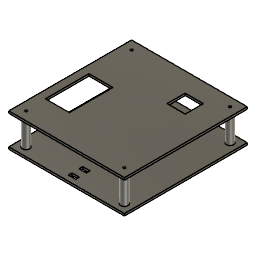
base_colonnine_M3_asole_aperture_superiori_Arduino_pacco_batteria (Autodesk Fusion 360 design; units mm, degrees)
part number: 2026-07-13-17-16-51-748
part number: 2026-07-13-17-16-52-029
part number: 2026-07-13-17-16-52-072
Autodesk Fusion 360 part; units mm, degrees
sketch "Schizzo1" plane through (0, 0, 0) normal (0, 0, 1) x (1, 0, 0) in component "01_Piano_inferiore_con_colonnine_M3"
  line L0 (-80, -85) -> (80, -85)
  line L1 (80, -85) -> (80, 85)
  line L2 (80, 85) -> (-80, 85)
  line L3 (-80, 85) -> (-80, -85)
extrude "Estrusione_Piano_inferiore" add sketch "Schizzo1" along normal blind 3 makes body 1 in component "01_Piano_inferiore_con_colonnine_M3"
ref_plane "Piano di lavoro1" through (0, 0, 43) normal (0, 0, 1) x (1, 0, 0) in component "02_Piano_superiore"
sketch "Schizzo1 (2)" plane through (0, 0, 43) normal (0, 0, 1) x (1, 0, 0) in component "02_Piano_superiore"
  line L0 (-80, -85) -> (80, -85)
  line L1 (80, -85) -> (80, 85)
  line L2 (80, 85) -> (-80, 85)
  line L3 (-80, 85) -> (-80, -85)
extrude "Estrusione_Piano_superiore" add sketch "Schizzo1 (2)" along normal blind 3 separate body makes body 2 in component "02_Piano_superiore"
ref_plane "Piano di lavoro1" through (0, 0, 3) normal (0, 0, 1) x (1, 0, 0) in component "01_Piano_inferiore_con_colonnine_M3"
ref_plane "Piano di lavoro2" through (0, 0, 40.4) normal (0, 0, 1) x (1, 0, 0) in component "01_Piano_inferiore_con_colonnine_M3"
sketch "Schizzo2" plane through (0, 0, 0) normal (0, 0, 1) x (1, 0, 0) in component "01_Piano_inferiore_con_colonnine_M3"
  line L0 (-5, -77.5) -> (5, -77.5)
  line L1 (5, -77.5) -> (5, -72.5)
  line L2 (5, -72.5) -> (-5, -72.5)
  line L3 (-5, -72.5) -> (-5, -77.5)
extrude "Asola_fascetta_01" cut sketch "Schizzo2" along normal blind 3 bodies 1 in component "01_Piano_inferiore_con_colonnine_M3"
sketch "Schizzo3" plane through (0, 0, 0) normal (0, 0, 1) x (1, 0, 0) in component "01_Piano_inferiore_con_colonnine_M3"
  line L0 (-5, -62.5) -> (5, -62.5)
  line L1 (5, -62.5) -> (5, -57.5)
  line L2 (5, -57.5) -> (-5, -57.5)
  line L3 (-5, -57.5) -> (-5, -62.5)
extrude "Asola_fascetta_02" cut sketch "Schizzo3" along normal blind 3 bodies 1 in component "01_Piano_inferiore_con_colonnine_M3"
sketch "Schizzo4" plane through (0, 0, 0) normal (0, 0, 1) x (1, 0, 0) in component "01_Piano_inferiore_con_colonnine_M3"
  line L0 (-5, -12.5) -> (5, -12.5)
  line L1 (5, -12.5) -> (5, -7.5)
  line L2 (5, -7.5) -> (-5, -7.5)
  line L3 (-5, -7.5) -> (-5, -12.5)
extrude "Asola_fascetta_03" cut sketch "Schizzo4" along normal blind 3 bodies 1 in component "01_Piano_inferiore_con_colonnine_M3"
sketch "Schizzo5" plane through (0, 0, 0) normal (0, 0, 1) x (1, 0, 0) in component "01_Piano_inferiore_con_colonnine_M3"
  line L0 (-5, 2.5) -> (5, 2.5)
  line L1 (5, 2.5) -> (5, 7.5)
  line L2 (5, 7.5) -> (-5, 7.5)
  line L3 (-5, 7.5) -> (-5, 2.5)
extrude "Asola_fascetta_04" cut sketch "Schizzo5" along normal blind 3 bodies 1 in component "01_Piano_inferiore_con_colonnine_M3"
sketch "Schizzo2 (2)" plane through (0, 0, 43) normal (0, 0, 1) x (1, 0, 0) in component "02_Piano_superiore"
  circle A0 centre (-68, -73) radius 1.6
extrude "Foro_M3_superiore_01" cut sketch "Schizzo2 (2)" along normal blind 3 bodies 2 in component "02_Piano_superiore"
sketch "Schizzo6" plane through (0, 0, 3) normal (0, 0, 1) x (1, 0, 0) in component "01_Piano_inferiore_con_colonnine_M3"
  circle A0 centre (-68, -73) radius 5
extrude "Estrusione_Colonnina_M3_01" add sketch "Schizzo6" along normal blind 40 bodies 1 in component "01_Piano_inferiore_con_colonnine_M3"
sketch "Schizzo7" plane through (0, 0, 0) normal (0, 0, 1) x (1, 0, 0) in component "01_Piano_inferiore_con_colonnine_M3"
  circle A0 centre (-68, -73) radius 1.6
extrude "Foro_passante_M3_colonnina_01" cut sketch "Schizzo7" along normal blind 43 bodies 1 in component "01_Piano_inferiore_con_colonnine_M3"
sketch "Schizzo8" plane through (0, 0, 40.4) normal (0, 0, 1) x (1, 0, 0) in component "01_Piano_inferiore_con_colonnine_M3"
  line L0 (-65.1, -71.3257) -> (-68, -69.6514)
  line L1 (-68, -69.6514) -> (-70.9, -71.3257)
  line L2 (-70.9, -71.3257) -> (-70.9, -74.6743)
  line L3 (-70.9, -74.6743) -> (-68, -76.3486)
  line L4 (-68, -76.3486) -> (-65.1, -74.6743)
  line L5 (-65.1, -74.6743) -> (-65.1, -71.3257)
extrude "Sede_dado_M3_01" cut sketch "Schizzo8" along normal blind 2.6 bodies 1 in component "01_Piano_inferiore_con_colonnine_M3"
sketch "Schizzo3 (2)" plane through (0, 0, 43) normal (0, 0, 1) x (1, 0, 0) in component "02_Piano_superiore"
  circle A0 centre (68, -73) radius 1.6
extrude "Foro_M3_superiore_02" cut sketch "Schizzo3 (2)" along normal blind 3 bodies 2 in component "02_Piano_superiore"
sketch "Schizzo9" plane through (0, 0, 3) normal (0, 0, 1) x (1, 0, 0) in component "01_Piano_inferiore_con_colonnine_M3"
  circle A0 centre (68, -73) radius 5
extrude "Estrusione_Colonnina_M3_02" add sketch "Schizzo9" along normal blind 40 bodies 1 in component "01_Piano_inferiore_con_colonnine_M3"
sketch "Schizzo10" plane through (0, 0, 0) normal (0, 0, 1) x (1, 0, 0) in component "01_Piano_inferiore_con_colonnine_M3"
  circle A0 centre (68, -73) radius 1.6
extrude "Foro_passante_M3_colonnina_02" cut sketch "Schizzo10" along normal blind 43 bodies 1 in component "01_Piano_inferiore_con_colonnine_M3"
sketch "Schizzo11" plane through (0, 0, 40.4) normal (0, 0, 1) x (1, 0, 0) in component "01_Piano_inferiore_con_colonnine_M3"
  line L0 (70.9, -71.3257) -> (68, -69.6514)
  line L1 (68, -69.6514) -> (65.1, -71.3257)
  line L2 (65.1, -71.3257) -> (65.1, -74.6743)
  line L3 (65.1, -74.6743) -> (68, -76.3486)
  line L4 (68, -76.3486) -> (70.9, -74.6743)
  line L5 (70.9, -74.6743) -> (70.9, -71.3257)
extrude "Sede_dado_M3_02" cut sketch "Schizzo11" along normal blind 2.6 bodies 1 in component "01_Piano_inferiore_con_colonnine_M3"
sketch "Schizzo4 (2)" plane through (0, 0, 43) normal (0, 0, 1) x (1, 0, 0) in component "02_Piano_superiore"
  circle A0 centre (68, 73) radius 1.6
extrude "Foro_M3_superiore_03" cut sketch "Schizzo4 (2)" along normal blind 3 bodies 2 in component "02_Piano_superiore"
sketch "Schizzo12" plane through (0, 0, 3) normal (0, 0, 1) x (1, 0, 0) in component "01_Piano_inferiore_con_colonnine_M3"
  circle A0 centre (68, 73) radius 5
extrude "Estrusione_Colonnina_M3_03" add sketch "Schizzo12" along normal blind 40 bodies 1 in component "01_Piano_inferiore_con_colonnine_M3"
sketch "Schizzo13" plane through (0, 0, 0) normal (0, 0, 1) x (1, 0, 0) in component "01_Piano_inferiore_con_colonnine_M3"
  circle A0 centre (68, 73) radius 1.6
extrude "Foro_passante_M3_colonnina_03" cut sketch "Schizzo13" along normal blind 43 bodies 1 in component "01_Piano_inferiore_con_colonnine_M3"
sketch "Schizzo14" plane through (0, 0, 40.4) normal (0, 0, 1) x (1, 0, 0) in component "01_Piano_inferiore_con_colonnine_M3"
  line L0 (70.9, 74.6743) -> (68, 76.3486)
  line L1 (68, 76.3486) -> (65.1, 74.6743)
  line L2 (65.1, 74.6743) -> (65.1, 71.3257)
  line L3 (65.1, 71.3257) -> (68, 69.6514)
  line L4 (68, 69.6514) -> (70.9, 71.3257)
  line L5 (70.9, 71.3257) -> (70.9, 74.6743)
extrude "Sede_dado_M3_03" cut sketch "Schizzo14" along normal blind 2.6 bodies 1 in component "01_Piano_inferiore_con_colonnine_M3"
sketch "Schizzo5 (2)" plane through (0, 0, 43) normal (0, 0, 1) x (1, 0, 0) in component "02_Piano_superiore"
  circle A0 centre (-68, 73) radius 1.6
extrude "Foro_M3_superiore_04" cut sketch "Schizzo5 (2)" along normal blind 3 bodies 2 in component "02_Piano_superiore"
sketch "Schizzo15" plane through (0, 0, 3) normal (0, 0, 1) x (1, 0, 0) in component "01_Piano_inferiore_con_colonnine_M3"
  circle A0 centre (-68, 73) radius 5
extrude "Estrusione_Colonnina_M3_04" add sketch "Schizzo15" along normal blind 40 bodies 1 in component "01_Piano_inferiore_con_colonnine_M3"
sketch "Schizzo16" plane through (0, 0, 0) normal (0, 0, 1) x (1, 0, 0) in component "01_Piano_inferiore_con_colonnine_M3"
  circle A0 centre (-68, 73) radius 1.6
extrude "Foro_passante_M3_colonnina_04" cut sketch "Schizzo16" along normal blind 43 bodies 1 in component "01_Piano_inferiore_con_colonnine_M3"
sketch "Schizzo17" plane through (0, 0, 40.4) normal (0, 0, 1) x (1, 0, 0) in component "01_Piano_inferiore_con_colonnine_M3"
  line L0 (-65.1, 74.6743) -> (-68, 76.3486)
  line L1 (-68, 76.3486) -> (-70.9, 74.6743)
  line L2 (-70.9, 74.6743) -> (-70.9, 71.3257)
  line L3 (-70.9, 71.3257) -> (-68, 69.6514)
  line L4 (-68, 69.6514) -> (-65.1, 71.3257)
  line L5 (-65.1, 71.3257) -> (-65.1, 74.6743)
extrude "Sede_dado_M3_04" cut sketch "Schizzo17" along normal blind 2.6 bodies 1 in component "01_Piano_inferiore_con_colonnine_M3"
sketch "Schizzo6 (2)" plane through (0, 0, 43) normal (0, 0, 1) x (1, 0, 0) in component "02_Piano_superiore"
  line L0 (20.83, 33.21) -> (45.83, 33.21)
  line L1 (45.83, 33.21) -> (45.83, 58.21)
  line L2 (45.83, 58.21) -> (20.83, 58.21)
  line L3 (20.83, 58.21) -> (20.83, 33.21)
extrude "Apertura_Arduino_25x25_D2_D7_S1_S8" cut sketch "Schizzo6 (2)" along normal blind 3 bodies 2 in component "02_Piano_superiore"
sketch "Schizzo7 (2)" plane through (0, 0, 43) normal (0, 0, 1) x (1, 0, 0) in component "02_Piano_superiore"
  line L0 (-69, -45) -> (-36, -45)
  line L1 (-36, -45) -> (-36, 15)
  line L2 (-36, 15) -> (-69, 15)
  line L3 (-69, 15) -> (-69, -45)
extrude "Apertura_pacco_batteria_PCB_cannone_60x33" cut sketch "Schizzo7 (2)" along normal blind 3 bodies 2 in component "02_Piano_superiore"
component "01_Piano_inferiore_con_colonnine_M3" placed x (1, 0, 0) y (0, 1, 0) z (0, 0, 1) at (0, 0, 0)
component "02_Piano_superiore" placed x (1, 0, 0) y (0, 1, 0) z (0, 0, 1) at (0, 0, 0)
equation "piano_inf_lunghezza = 170.0 mm" comment "Piano inferiore"
equation "piano_inf_larghezza = 160.0 mm" comment "Piano inferiore"
equation "piano_inf_spessore = 3.0 mm" comment "Piano inferiore"
equation "d4 = piano_inf_spessore"
equation "distanza_piani = 40.0 mm" comment "Luce libera fra i piani"
equation "piano_sup_lunghezza = 170.0 mm" comment "Piano superiore"
equation "piano_sup_larghezza = 160.0 mm" comment "Piano superiore"
equation "piano_sup_spessore = 3.0 mm" comment "Piano superiore"
equation "colonnina_diametro = 10.0 mm" comment "Colonnine base"
equation "foro_vite_M3 = 3.2 mm" comment "Gioco vite M3"
equation "colonnina_offset_bordo = 12.0 mm" comment "Centro colonnina dal bordo"
equation "dado_M3_chiave = 5.8 mm" comment "Sede esagonale dado M3"
equation "dado_M3_profondita = 2.6 mm" comment "Profondita sede dado M3"
equation "d15 = piano_inf_spessore + distanza_piani"
equation "d17 = piano_sup_spessore"
equation "d19 = piano_inf_spessore"
equation "d21 = piano_inf_spessore + distanza_piani - dado_M3_profondita"
equation "asola_fascetta_lunghezza = 10.0 mm" comment "Asola fascetta, asse Est-Ovest"
equation "asola_fascetta_larghezza = 5.0 mm" comment "Asola fascetta, asse Sud-Nord"
equation "d25 = piano_inf_spessore"
equation "d27 = piano_inf_spessore"
equation "d29 = piano_inf_spessore"
equation "d31 = piano_inf_spessore"
equation "d33 = piano_sup_spessore"
equation "d35 = distanza_piani"
equation "d37 = piano_inf_spessore + distanza_piani"
equation "d39 = dado_M3_profondita"
equation "d41 = piano_sup_spessore"
equation "d43 = distanza_piani"
equation "d45 = piano_inf_spessore + distanza_piani"
equation "d47 = dado_M3_profondita"
equation "d49 = piano_sup_spessore"
equation "d51 = distanza_piani"
equation "d53 = piano_inf_spessore + distanza_piani"
equation "d55 = dado_M3_profondita"
equation "d57 = piano_sup_spessore"
equation "d59 = distanza_piani"
equation "d61 = piano_inf_spessore + distanza_piani"
equation "d63 = dado_M3_profondita"
equation "apertura_arduino_larghezza = 25.0 mm" comment "Apertura superiore sopra Arduino"
equation "apertura_arduino_lunghezza = 25.0 mm" comment "Apertura superiore sopra Arduino"
equation "apertura_arduino_centro_x = 33.33 mm" comment "Centro Est-Ovest apertura Arduino"
equation "apertura_arduino_centro_y = 45.71 mm" comment "Centro Sud-Nord apertura Arduino"
equation "apertura_pacco_batteria_larghezza = 33.0 mm" comment "Apertura superiore pacco batteria PCB cannone"
equation "apertura_pacco_batteria_lunghezza = 60.0 mm" comment "Apertura superiore pacco batteria PCB cannone"
equation "apertura_pacco_batteria_centro_x = -52.5 mm" comment "Centro Est-Ovest apertura pacco batteria PCB cannone"
equation "apertura_pacco_batteria_centro_y = -15.0 mm" comment "Centro Sud-Nord apertura pacco batteria PCB cannone"
equation "d73 = piano_sup_spessore"
equation "d75 = piano_sup_spessore"
named bodies: "Piano_inferiore_con_colonnine_M3", "Piano_superiore"
